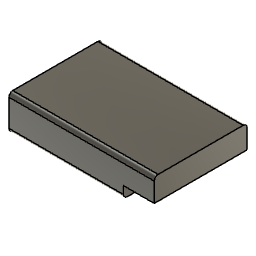
Qwiic_USB_Bridge_3DP v28 (Autodesk Fusion 360 archive; units mm, degrees)
design "USB_A_SMT_Mechanical"
Autodesk Fusion 360 part; units mm, degrees
sketch "Sketch1" plane through (0, 0, 0) normal (1, 0, 0) x (0, 1, 0)
  line L0 (5.5, 2.25) -> (-5.5, 2.25)
  line L1 (-6, 1.75) -> (-6, -1.75)
  line L2 (-5.5, -2.25) -> (5.5, -2.25)
  line L3 (6, -1.75) -> (6, 1.75)
  line L4 (6, 2.25) -> (-6, -2.25) construction
  line L5 (-6, 2.25) -> (6, -2.25) construction
  arc A0 (-5.5, 2.25) -> (-6, 1.75) centre (-5.5, 1.75) ccw
  arc A1 (-6, -1.75) -> (-5.5, -2.25) centre (-5.5, -1.75) ccw
  arc A2 (6, 1.75) -> (5.5, 2.25) centre (5.5, 1.75) ccw
  arc A3 (5.5, -2.25) -> (6, -1.75) centre (5.5, -1.75) ccw
  dimension "d1" = 12
  dimension "d2" = 4.5
  dimension "d3" = 0.5
  dimension "d4" = 0.5
  dimension "d5" = 0.5
  dimension "d6" = 0.5
  constraint horizontal L0
  constraint perpendicular L0 L1
  constraint parallel L0 L2
  constraint parallel L1 L3
  constraint coincident L4 origin
  constraint coincident L5 origin
  constraint coincident L5.start L0
  constraint coincident L5.start L1
  constraint tangent L0 A0
  constraint tangent L1 A0
  constraint coincident L4.end L1
  constraint coincident L4.end L2
  constraint tangent L1 A1
  constraint tangent L2 A1
  constraint coincident L4.start L0
  constraint coincident L4.start L3
  constraint tangent L0 A2
  constraint tangent L3 A2
  constraint coincident L5.end L2
  constraint coincident L5.end L3
  constraint tangent L2 A3
  constraint tangent L3 A3
  measures "d1" distance of L4.end L5.end
  measures "d2" distance of L5.start L4.end
  measures "d3" radius of A0
  measures "d4" radius of A1
  measures "d5" radius of A2
  measures "d6" radius of A3
extrude "Extrude1" add sketch "Sketch1" along normal blind 18.8
sketch "Sketch2" plane through (18.8, 0, 0) normal (1, 0, 0) x (0, 1, 0)
  arc A0 (5.5, -2.25) -> (6, -1.75) centre (5.5, -1.75) ccw
  line L0 (6, -1.75) -> (6, 1.75)
  arc A1 (6, 1.75) -> (5.5, 2.25) centre (5.5, 1.75) ccw
  line L1 (5.5, 2.25) -> (-5.5, 2.25)
  arc A2 (-5.5, 2.25) -> (-6, 1.75) centre (-5.5, 1.75) ccw
  line L2 (-6, 1.75) -> (-6, -1.75)
  arc A3 (-6, -1.75) -> (-5.5, -2.25) centre (-5.5, -1.75) ccw
  line L3 (-5.5, -2.25) -> (5.5, -2.25)
  line L4 (0, 2.25) -> (0, -0.75)
  line L5 (0, -0.75) -> (6, -0.75)
  line L6 (6, -0.75) -> (6, -2.25)
  line L7 (6, -2.25) -> (0, -2.25)
  line L8 (0, -2.25) -> (0, -0.75)
  line L9 (0, -0.75) -> (-6, -0.75)
  line L10 (-6, -0.75) -> (-6, -2.25)
  line L11 (-6, -2.25) -> (0, -2.25)
  line L12 (0, -2.25) -> (0, -0.75)
  dimension "d9" = 3
  constraint midpoint L1 L4.start
  constraint perpendicular L1 L4
  constraint horizontal L5
  constraint vertical L6
  constraint horizontal L7
  constraint vertical L8
  constraint horizontal L9
  constraint vertical L10
  constraint horizontal L11
  constraint vertical L12
  measures "d9" distance of L4.start L4.end
extrude "Extrude2" cut sketch "Sketch2" against normal blind 4 contours A0 L0 L3 L5 L6 L7 L8 L12 | L2 A3 L3 L8 L9 L10 L11 L12
